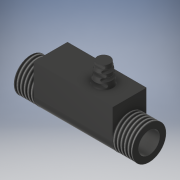
# Autodesk Inventor part: 0.375 IN Flow Meter  SEN-206F
Saved by Autodesk Inventor 2019 (Build 230136000, 136)
## iProperties
Created: 2020-10-03
Part Number: 0.375 IN Flow Meter  SEN-206F
Material: Polypropylene
Document SubType Name: Modeling
Designer: J. LENDI
Mass: 12.9077 g
Surface Area: 69.7677 cm^2
Volume: 14.3578 cm^3
Density: 0.899 g/cm^3
Appearance: Smooth - Black
Author: J. LENDI
Autodesk Inventor part; units mm, degrees
ref_plane "YZ Plane" through (0, 0, 0) normal (1, 0, 0) x (0, 1, 0)
ref_plane "XZ Plane" through (0, 0, 0) normal (0, 1, 0) x (-1, 0, 0)
ref_plane "XY Plane" through (0, 0, 0) normal (0, 0, 1) x (1, 0, 0)
sketch "Sketch1" plane through (0, 0, 0) normal (1, 0, 0) x (0, 1, 0)
  line L0 (-11.7475, 8.5725) -> (11.7475, 8.5725)
  line L1 (11.7475, 8.5725) -> (11.7475, -8.5725)
  line L2 (11.7475, -8.5725) -> (-11.7475, -8.5725)
  line L3 (-11.7475, -8.5725) -> (-11.7475, 8.5725)
  line L4 (-11.7475, 8.5725) -> (11.7475, -8.5725) construction
  line L5 (11.7475, 8.5725) -> (-11.7475, -8.5725) construction
  circle A0 centre (-3.175, 0) radius 8.5725 construction
  circle A1 centre (-3.175, 0) radius 5.3975
  point P0 (0, 0)
  dimension "d0" = 17.145
  dimension "d1" = 23.495
  dimension "d2" = 17.145
  dimension "d3" = 8.5725
  dimension "d4" = 10.795
  constraints: 12 end point, 2 centre point, 2 midpoint, 2 parallel, 1 coincident, 1 horizontal, 1 perpendicular, 1 tangent
  measures "d0" distance between parallel lines of L2 L0
  measures "d1" distance between parallel lines of L3 L1
  measures "d2" diameter of A0
  measures "d3" distance from line of L0 A0.centre
  measures "d4" diameter of A1
extrude "Extrusion1" add sketch "Sketch1" along normal mid plane 40
sketch "Sketch2" plane through (20, 0, 0) normal (1, 0, 0) x (0, 0, -1)
  circle A0 centre (0, -3.175) radius 5.3975 projected
  circle A1 centre (0, -3.175) radius 8.5725
  line L0 (-8.5725, -11.7475) -> (8.5725, -11.7475) projected
  point P0 (0, 0)
  constraints: 1 centre point, 1 coincident, 1 tangent
extrude "Extrusion2" add sketch "Sketch2" along normal blind 10
thread "Thread1" size "3/4" designation "3/4 - 14 NPT" standard "NPT for PVC Pipe and Fitting" length 20.1676
mirror "Mirror1" about plane through (0, 0, 0) normal (1, 0, 0) of "Extrusion2"
fillet "Fillet2" radius 8.509 2 edges at (0, -11.7475, -8.5725) (0, -11.7475, 8.5725)
sketch "Sketch3" plane through (-20, 11.7475, 8.5725) normal (0, 1, 0) x (1, 0, 0)
  line L0 (0, 8.509) -> (40, 8.509) projected
  circle A0 centre (27, 8.509) radius 4.7625
  line L1 (40, 17.145) -> (40, 0) projected
  point P0 (20, 8.5725)
  dimension "d13" = 9.525
  dimension "d14" = 13
  constraints: 1 centre point, 1 point on line
  measures "d13" diameter of A0
  measures "d14" distance from line of A0.centre L1
ref_plane "Work Plane1" through (-20, 21.7475, 8.5725) normal (0, 1, 0) x (1, 0, 0)
sketch "Sketch4" plane through (-20, 21.7475, 8.5725) normal (0, 1, 0) x (1, 0, 0)
  line L0 (0, 8.509) -> (40, 8.509) projected
  circle A0 centre (27, 8.509) radius 3.175
  circle A1 centre (27, 8.509) radius 4.7625 construction
  line L1 (40, 17.145) -> (40, 0) projected
  point P0 (20, 8.5725)
  dimension "d16" = 6.35
  dimension "d17" = 13
  constraints: 1 centre point, 1 point on line
  measures "d16" diameter of A0
  measures "d17" distance from line of L1 A0.centre
loft "Loft1" add profiles "Sketch4", "Sketch3"
ref_plane "Work Plane2" through (20, -3.175, 8.5725) normal (0, 0, 1) x (1, 0, 0)
sketch "Sketch5" plane through (20, -3.175, 8.5725) normal (0, 0, 1) x (1, 0, 0)
  line L0 (-16.175, 24.9225) -> (-9.825, 24.9225) construction
  line L1 (-17.7625, 14.9225) -> (-8.2375, 14.9225) construction
  line L2 (-17.7625, 14.9225) -> (-16.175, 24.9225) construction
  line L3 (-17.7625, 18.0975) -> (-15.6987, 18.0975)
  line L4 (-17.7625, 19.685) -> (-15.6987, 19.685)
  line L5 (-14.905, 24.9225) -> (-14.905, 14.9225) construction
  line L6 (0, 14.9225) -> (-40, 14.9225) projected
  line L7 (-16.175, 24.9225) -> (-9.825, 24.9225) projected
  line L8 (-11.095, 24.9225) -> (-11.095, 14.9225) construction
  line L9 (-15.6987, 18.0975) -> (-15.6987, 19.685) construction
  arc A0 (-15.6987, 18.0975) -> (-15.6987, 19.685) centre (-15.6987, 18.8913) ccw
  line L10 (-13, 24.9225) -> (-13, 14.9225) construction
  line L11 (-17.7625, 22.86) -> (-15.6987, 22.86)
  arc A1 (-15.6987, 21.2725) -> (-15.6987, 22.86) centre (-15.6987, 22.0663) ccw
  line L12 (-15.6987, 21.2725) -> (-15.6987, 22.86) construction
  line L13 (-17.7625, 21.2725) -> (-15.6987, 21.2725)
  line L14 (-8.2375, 14.9225) -> (-9.825, 24.9225) construction
  line L15 (-8.2375, 18.0975) -> (-10.3013, 18.0975)
  line L16 (-8.2375, 19.685) -> (-10.3013, 19.685)
  line L17 (-10.3013, 18.0975) -> (-10.3013, 19.685) construction
  arc A2 (-10.3013, 19.685) -> (-10.3013, 18.0975) centre (-10.3013, 18.8913) ccw
  line L18 (-8.2375, 22.86) -> (-10.3013, 22.86)
  arc A3 (-10.3013, 22.86) -> (-10.3013, 21.2725) centre (-10.3013, 22.0663) ccw
  line L19 (-10.3013, 21.2725) -> (-10.3013, 22.86) construction
  line L20 (-8.2375, 21.2725) -> (-10.3013, 21.2725)
  line L21 (-17.7625, 18.0975) -> (-17.7625, 19.685)
  line L22 (-17.7625, 21.2725) -> (-17.7625, 22.86)
  line L23 (-8.2375, 18.0975) -> (-8.2375, 19.685)
  line L24 (-8.2375, 21.2725) -> (-8.2375, 22.86)
  point P0 (-20, 3.175)
  point P1 (-17.7625, 24.9225)
  point P2 (-17.7625, 14.9225)
  point P3 (-8.2375, 24.9225)
  point P4 (-8.2375, 14.9225)
  dimension "d22" = 1.5875
  dimension "d23" = 3.175
  dimension "d25" = 3.81
  dimension "d26" = 6.35
  dimension "d27" = 1.27
  dimension "d38" = 3.175
  constraints: 40 end point, 14 symmetric about line, 8 point on circle, 8 point on line, 4 centre point, 4 vertical, 3 perpendicular, 2 tangent, 1 horizontal, 1 midpoint, 11 other
  measures "d22" distance between parallel lines of L3 L4
  measures "d23" distance between parallel lines of L1 L3
  measures "d25" distance between parallel lines of L8 L5
  measures "d26" distance of L0.start L0.end
  measures "d27" distance from line of L5 L2.end
  measures "d38" distance of L11.start L4.start
extrude "Extrusion3" cut sketch "Sketch5" against normal through all
sketch "Sketch6" plane through (0, 0, 0) normal (1, 0, 0) x (0, 1, 0)
  line L0 (11.7475, -4.699) -> (21.7475, -3.1115) construction
  line L1 (21.7475, 3.2385) -> (21.7475, -3.1115) construction
  line L2 (11.7475, 4.826) -> (21.7475, 3.2385) construction
  line L3 (11.7475, 8.5725) -> (11.7475, -8.5725) construction
  line L4 (11.7475, 4.826) -> (11.7475, -4.699) projected
  line L5 (11.7475, 0.0635) -> (21.7475, 0.0635) construction
  line L6 (11.7475, 1.9685) -> (21.7475, 1.9685) construction
  line L7 (11.7475, -1.8415) -> (21.7475, -1.8415) construction
  line L8 (12.5412, -4.699) -> (12.5412, -2.6353)
  line L9 (12.5412, -2.6353) -> (14.1287, -2.6353) construction
  line L10 (14.1287, -2.6353) -> (14.1287, -4.699)
  arc A0 (14.1287, -2.6353) -> (12.5412, -2.6353) centre (13.335, -2.6353) ccw
  line L11 (14.9225, 3.3576) -> (14.9225, -3.2306) construction
  line L12 (16.51, -2.8977) -> (16.51, 3.0247) construction
  line L13 (18.0975, 2.6736) -> (18.0975, -2.5466) construction
  line L14 (19.685, -2.1689) -> (19.685, 2.2959) construction
  arc A1 (18.1165, -2.6353) -> (16.529, -2.6353) centre (17.3228, -2.6353) ccw
  line L15 (16.529, -2.6353) -> (18.1165, -2.6353) construction
  line L16 (16.529, -4.699) -> (16.529, -2.6353)
  line L17 (18.1165, -2.6353) -> (18.1165, -4.699)
  arc A2 (21.5455, -2.6353) -> (19.958, -2.6353) centre (20.7518, -2.6353) ccw
  line L18 (19.958, -4.699) -> (19.958, -2.6353)
  line L19 (21.5455, -2.6353) -> (21.5455, -4.699)
  line L20 (11.7475, 4.826) -> (21.7475, 3.2385) construction
  line L21 (21.7475, -3.1115) -> (21.7475, 3.2385) construction
  line L22 (12.5413, 4.826) -> (12.5412, 2.7622)
  line L23 (12.5412, 2.7622) -> (14.1287, 2.7622) construction
  line L24 (14.1287, 2.7622) -> (14.1288, 4.826)
  arc A3 (12.5412, 2.7622) -> (14.1287, 2.7622) centre (13.335, 2.7622) ccw
  line L25 (14.9225, -3.2306) -> (14.9225, 3.3576) construction
  line L26 (16.51, 3.0247) -> (16.51, -2.8977) construction
  line L27 (18.0975, -2.5466) -> (18.0975, 2.6736) construction
  arc A4 (16.529, 2.7622) -> (18.1165, 2.7622) centre (17.3228, 2.7622) ccw
  line L28 (16.529, 2.7622) -> (18.1165, 2.7622) construction
  line L29 (16.5291, 4.826) -> (16.529, 2.7622)
  line L30 (18.1165, 2.7622) -> (18.1166, 4.826)
  arc A5 (19.9581, 2.7622) -> (21.5455, 2.7622) centre (20.7518, 2.7622) ccw
  line L31 (19.9581, 4.826) -> (19.9581, 2.7622)
  line L32 (21.5455, 2.7622) -> (21.5456, 4.826)
  line L33 (19.958, -4.699) -> (21.5455, -4.699)
  line L34 (19.9581, 4.826) -> (21.5456, 4.826)
  line L35 (11.7475, 4.826) -> (14.1288, 4.826)
  line L36 (11.7475, 4.826) -> (14.1288, 4.826)
  line L37 (16.5291, 4.826) -> (18.1166, 4.826)
  line L38 (16.5291, 4.826) -> (18.1166, 4.826)
  line L39 (19.9581, 4.826) -> (21.5456, 4.826)
  line L40 (11.7475, -4.699) -> (14.1287, -4.699)
  line L41 (16.529, -4.699) -> (18.1165, -4.699)
  point P0 (0, 0)
  dimension "d45" = 3.81
  dimension "d46" = 1.905
  dimension "d47" = 1.5875
  dimension "d48" = 0.7937
  dimension "d49" = 3.175
  dimension "d52" = 3.9878
  dimension "d59" = 3.429
  constraints: 66 end point, 23 symmetric about line, 12 point on circle, 8 horizontal, 6 centre point, 6 perpendicular, 6 point on line, 3 tangent, 2 midpoint, 1 vertical, 20 other
  measures "d45" distance between parallel lines of L6 L7
  measures "d46" distance between parallel lines of L5 L7
  measures "d47" distance between parallel lines of L8 L10
  measures "d48" distance between parallel lines of L8 L4
  measures "d49" distance between parallel lines of L3 L11
  measures "d52" distance of A0.centre A1.centre
  measures "d59" distance of A1.centre A2.centre
extrude "Extrusion4" cut sketch "Sketch6" along normal through all
equation "\"d2\" = d0"
equation "\"d3\" = 0.5 * d0"
equation "\"d17\" = d14"
equation "\"d27\" = -0.5 * d25 + 0.5 * d26"
equation "\"d46\" = 0.5 * d45"
body "Solid1"
